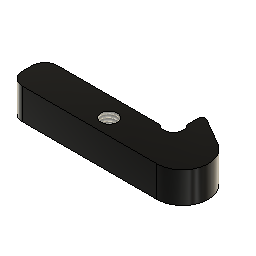
ThrowerLowerPlateHolder v4 (Autodesk Fusion 360 design; units mm, degrees)
Autodesk Fusion 360 part; units mm, degrees
sketch "Sketch1" plane through (0, 0, 0) normal (0, 0, 1) x (1, 0, 0)
  line L0 (0, 2.1213) -> (0, 3.934)
  line L1 (0.75, 4.367) -> (4.9119, 1.9641)
  line L2 (2.9119, -5.5) -> (-18, -5.5)
  line L3 (-20, -3.5) -> (-20, -2)
  line L4 (-18, 0) -> (-2.1213, 0)
  line L5 (0, 0) -> (-1.0607, 1.0607) construction
  arc A0 (-2.1213, 0) -> (0, 2.1213) centre (-1.0607, 1.0607) ccw
  arc A1 (0, 2.1213) -> (-2.1213, 0) centre (-1.0607, 1.0607) ccw construction
  line L6 (-2.1213, 0) -> (0, 0) construction
  line L7 (0, 0) -> (0, 2.1213) construction
  circle A2 centre (-7, -3) radius 1.5
  arc A3 (0.75, 4.367) -> (0, 3.934) centre (0.5, 3.934) ccw
  arc A4 (2.9119, -5.5) -> (4.9119, 1.9641) centre (2.9119, -1.5) ccw
  arc A5 (-18, 0) -> (-20, -2) centre (-18, -2) ccw
  arc A6 (-20, -3.5) -> (-18, -5.5) centre (-18, -3.5) ccw
  point P0 (0, 4.8)
  point P1 (-20, -5.5)
  point P2 (-20, 0)
  dimension "d1" = 4.8
  dimension "d2" = 20
  dimension "d3" = 5.5
  dimension "d4" = 30
  dimension "d5" = 1.5
  dimension "d6" = 45
  dimension "d7" = 3
  dimension "d8" = 3
  dimension "d10" = 0.5
  dimension "d11" = 4
  dimension "d12" = 2
  dimension "d13" = 2
  dimension "d16" = 7
  constraint coincident L5.start L6.end
  constraint vertical L0
  constraint perpendicular L0 L2
  constraint perpendicular L2 L3
  constraint perpendicular L3 L4
  constraint coincident L5.end A0.centre
  constraint coincident L5.start A0
  constraint concentric A0 A1
  constraint perpendicular L3 L6
  constraint vertical L7
  constraint coincident P0 L0
  constraint coincident P0 L1
  constraint tangent L0 A3
  constraint tangent L1 A3
  constraint tangent L1 A4
  constraint tangent L2 A4
  constraint coincident P2 L4
  constraint coincident P2 L3
  constraint tangent L4 A5
  constraint tangent L3 A5
  constraint coincident P1 L3
  constraint coincident P1 L2
  constraint tangent L3 A6
  constraint tangent L2 A6
  measures "d1" distance of L5.start P0
  measures "d2" distance of P2 L5.start
  measures "d3" distance of P1 P2
  measures "d4" angle of L1 L4
  measures "d5" distance of L5.start L5.end
  measures "d6" angle of L4 L5
  measures "d7" diameter of A2
  measures "d8" distance of L4 A2.centre
  measures "d10" radius of A3
  measures "d11" radius of A4
  measures "d12" radius of A5
  measures "d13" radius of A6
  measures "d16" distance of L0 A2.centre
extrude "Extrude1" add sketch "Sketch1" along normal blind 4.8
thread "Thread1" "ISO Metric profile 3.0 M3x0.5 6H" major diameter 3.086 minor diameter 2.529 pitch 0.5 angle 60 resizes the face on face at (-5.5019, -3.0748, 3.2)
